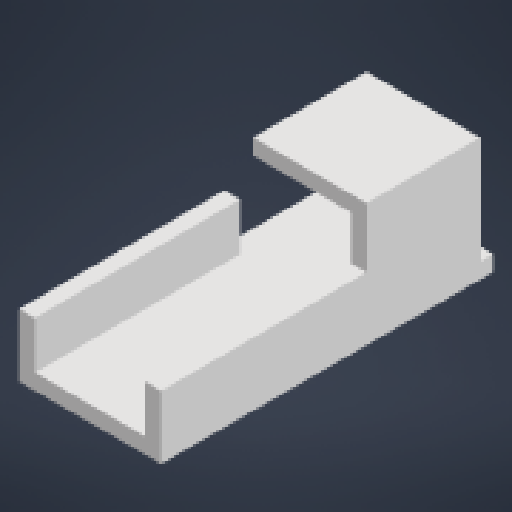
# Autodesk Inventor part: inslide
Saved by Autodesk Inventor 2026.2 (Build 302298000, 298)
## iProperties
Created: 2026-02-23
Part Number: inslide
Material: Generic
Document SubType Name: Sheet Metal
Designer: danda
Density: 1 g/cm^3
Sheet Metal Rule: Default_mm
Appearance: Default
Author: danda
Autodesk Inventor part; units mm, degrees
ref_plane "YZ Plane" through (0, 0, 0) normal (1, 0, 0) x (0, 1, 0)
ref_plane "XZ Plane" through (0, 0, 0) normal (0, 1, 0) x (-1, 0, 0)
ref_plane "XY Plane" through (0, 0, 0) normal (0, 0, 1) x (1, 0, 0)
sketch "Sketch1" plane through (0, 0, 0) normal (0, 0, 1) x (1, 0, 0)
  line L0 (13.7104, 12.7791) -> (48.7104, 12.7791)
  line L1 (48.7104, 12.7791) -> (48.7104, 27.7791)
  line L2 (13.7104, 12.7791) -> (13.7104, 27.7791)
  line L3 (8.7104, 27.7791) -> (8.7104, 7.7791)
  line L4 (8.7104, 7.7791) -> (53.7104, 7.7791)
  line L5 (53.7104, 7.7791) -> (53.7104, 27.7791)
  line L6 (8.7104, 27.7791) -> (13.7104, 27.7791)
  line L7 (48.7104, 27.7791) -> (53.7104, 27.7791)
  point P0 (0, 0)
  dimension "d0" = 35
  dimension "d1" = 15
  dimension "d2" = 15
  dimension "d3" = 5
  constraints: 16 end point, 3 horizontal, 2 perpendicular, 1 vertical, 2 other
  measures "d0" distance of L0.start L0.end
  measures "d1" distance of L0.end L1.end
  measures "d2" distance of L0.start L2.end
  measures "d3" distance between parallel lines of L2 L3
extrude "Extrusion1" add sketch "Sketch1" along normal blind 100 and the other way blind 5
sketch "Sketch2" plane through (8.7104, 7.7791, -5) normal (0, -1, 0) x (1, 0, 0)
  circle A0 centre (39.17, 93.8) radius 2.5
  line L0 (45, 0) -> (45, 105) projected
  line L1 (0, 105) -> (45, 105) projected
  point P0 (-8.7104, 5)
  dimension "d6" = 5
  dimension "d7" = 5.83
  dimension "d8" = 11.2
  constraints: 1 centre point
  measures "d6" diameter of A0
  measures "d7" distance from line of L0 A0.centre
  measures "d8" distance from line of L1 A0.centre
extrude "Extrusion2" cut sketch "Sketch2" against normal blind 2
sketch "Sketch3" plane through (8.7104, 7.7791, 100) normal (-1, 0, 0) x (0, 0, 1)
  line L0 (-105, 20) -> (-105, 5) projected
  line L1 (-105, 5) -> (0, 5) projected
  line L2 (-105, 20) -> (-105, 5)
  line L3 (-105, 5) -> (-65, 5)
  line L4 (-65, 5) -> (-65, 20)
  line L5 (-65, 20) -> (-105, 20)
  point P0 (-100, -7.7791)
  dimension "d13" = 40
  constraints: 8 end point, 2 perpendicular, 1 point on line, 1 vertical
  measures "d13" distance of L0.end L3.end
extrude "Extrusion3" cut sketch "Sketch3" against normal blind 10
sketch "Sketch4" plane through (0, 0, -5) normal (0, 0, -1) x (-1, 0, 0)
  line L0 (-53.7104, 27.7791) -> (-53.7104, 7.7791) projected
  line L1 (-53.7104, 7.7791) -> (-8.7104, 7.7791)
  line L2 (-17.7104, 42.7791) -> (-17.7104, 46.7534)
  line L3 (-17.7104, 46.7534) -> (-53.7104, 46.7534)
  line L4 (-53.7104, 46.7534) -> (-53.7104, 7.7791)
  line L5 (-48.7104, 12.7791) -> (-13.7104, 12.7791)
  line L6 (-10.7104, 42.7791) -> (-10.7104, 41.7534)
  line L7 (-10.7104, 41.7534) -> (-48.7104, 41.7534)
  line L8 (-48.7104, 41.7534) -> (-48.7104, 12.7791)
  line L9 (-17.7104, 42.7791) -> (-10.7104, 42.7791)
  line L10 (-8.7104, 12.7791) -> (-13.7104, 12.7791) projected
  line L11 (-13.7104, 12.7791) -> (-8.7104, 12.7791)
  line L12 (-8.7104, 12.7791) -> (-8.7104, 7.7791)
  line L13 (-17.7104, 42.7791) -> (-17.7104, 41.7534)
  point P0 (0, 0)
  point P1 (-17.7104, 44.7534)
  dimension "d16" = 36
  dimension "d17" = 40
  dimension "d18" = 5
  dimension "d19" = 30
  constraints: 24 end point, 5 perpendicular, 4 parallel, 2 horizontal, 1 point on line, 1 other
  measures "d16" distance of L3.end L2.end
  measures "d17" distance of L2.end L1.end
  measures "d18" distance between parallel lines of L4 L8
  measures "d19" distance between parallel lines of L5 L9
extrude "Extrusion4" add sketch "Sketch4" against normal blind 40 contours L4 L3 L2 L13 L7 L8 L5 L10 L12 L1 L0
extrude "Extrusion5" cut sketch "Sketch4" against normal blind 4
sketch "Sketch5" plane through (0, 0, -1) normal (0, 0, -1) x (-1, 0, 0)
  line L0 (-8.7104, 12.7791) -> (-13.7104, 12.7791) projected
  line L1 (-48.7104, 41.7534) -> (-48.7104, 12.7791) projected
  line L2 (-8.7104, 12.7791) -> (-8.7104, 7.7791) projected
  line L3 (-8.7104, 12.7791) -> (-8.7104, 7.7791)
  line L4 (-8.7104, 7.7791) -> (-53.7104, 7.7791) projected
  line L5 (-8.7104, 7.7791) -> (-53.7104, 7.7791)
  line L6 (-53.7104, 7.7791) -> (-53.7104, 12.7791)
  line L7 (-53.7104, 12.7791) -> (-8.7104, 12.7791)
  point P0 (0, 0)
  point P1 (-10.7104, 9.7791)
  constraints: 8 end point, 3 perpendicular, 1 vertical
extrude "Extrusion6" add sketch "Sketch5" along normal blind 4
equation "\"BendRadius\" = Thickness"
equation "\"BendReliefWidth\" = Thickness"
equation "\"BendReliefDepth\" = 0.5 * Thickness"
equation "\"CornerReliefSize\" = 4 * Thickness"
equation "\"MinimumRemnant\" = 2 * Thickness"
equation "\"TransitionRadius\" = BendRadius"
equation "\"JacobiRadiusSize\" = BendRadius"
equation "\"GapSize\" = Thickness"
equation "\"Thickness\" = 0.5"
body "Solid1"
